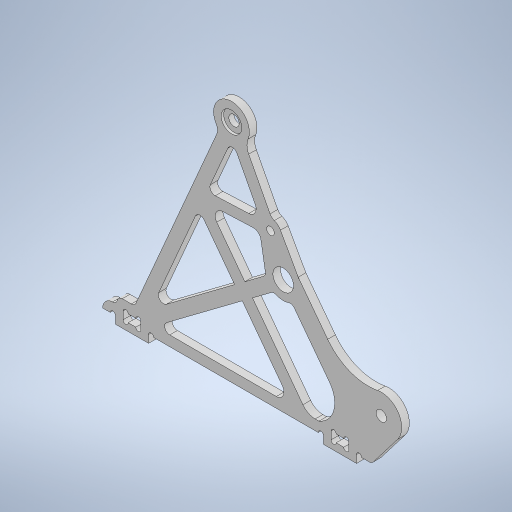
# Autodesk Inventor part: 左フレーム
Saved by Autodesk Inventor 2023 (Build 270158000, 158)
## iProperties
Created: 2022-04-10
Part Number: 左フレーム
Material: Generic
Document SubType Name: Modeling
Designer: acps
Density: 1 g/cm^3
Appearance: Default
Author: acps
Autodesk Inventor part; units mm, degrees
ref_plane "YZ Plane" through (0, 0, 0) normal (1, 0, 0) x (0, 1, 0)
ref_plane "XZ Plane" through (0, 0, 0) normal (0, 1, 0) x (-1, 0, 0)
ref_plane "XY Plane" through (0, 0, 0) normal (0, 0, 1) x (1, 0, 0)
sketch "Sketch1" plane through (0, 0, 0) normal (0, 0, 1) x (1, 0, 0)
  circle A0 centre (76.7566, -3) radius 1
  circle A1 centre (71.7566, -3) radius 1
  circle A2 centre (71.7566, -6) radius 1
  circle A3 centre (-4.7865, -3) radius 1
  circle A4 centre (-4.7865, -6) radius 1
  circle A5 centre (-9.7865, -6) radius 1
  circle A6 centre (-9.7865, -3) radius 1
  circle A7 centre (76.7566, -6) radius 1
  circle A8 centre (31.7211, 82.4471) radius 2.025
  circle A9 centre (31.7211, 82.4471) radius 7
  circle A10 centre (47, 53.101) radius 1.5
  circle A11 centre (52, 38.9589) radius 4.025
  circle A12 centre (52, 38.9589) radius 7.025
  circle A13 centre (47, 53.101) radius 4.5
  circle A14 centre (90.4665, 12.0244) radius 2.025
  circle A15 centre (66.7566, -6) radius 1
  circle A16 centre (81.7566, -6) radius 1
  line L0 (67.7566, -9) -> (80.7566, -9)
  line L1 (80.7566, -9) -> (80.7566, -6)
  line L2 (67.7566, -6) -> (67.7566, -9)
  circle A17 centre (-14.7865, -6) radius 1
  line L3 (-13.7865, -6) -> (-13.7865, -9)
  line L4 (-13.7865, -9) -> (-0.7865, -9)
  circle A18 centre (0.2135, -6) radius 1
  line L5 (-0.7865, -9) -> (-0.7865, -6)
  line L6 (72.7566, -3) -> (75.7566, -3)
  line L7 (70.7566, -3) -> (70.7566, -6)
  line L8 (77.7566, -3) -> (77.7566, -6)
  line L9 (72.7566, -6) -> (75.7566, -6)
  line L10 (67.7566, -6) -> (70.7566, -6)
  line L11 (77.7566, -6) -> (80.7566, -6)
  line L12 (1.2135, -6) -> (65.7566, -6)
  line L13 (-8.7865, -3) -> (-5.7865, -3)
  line L14 (-3.7865, -3) -> (-3.7865, -6)
  line L15 (-10.7865, -3) -> (-10.7865, -6)
  line L16 (-13.7865, -6) -> (-10.7865, -6)
  line L17 (-3.7865, -6) -> (-0.7865, -6)
  line L18 (-5.7865, -6) -> (-8.7865, -6)
  arc A19 (-14.9185, -2.0022) -> (-18.7865, -6) centre (-14.7865, -6) ccw
  line L19 (-15.7865, -6) -> (-18.7865, -6)
  arc A20 (-14.9185, -2.0022) -> (-13.0476, -0.5016) centre (-14.9845, -0.0033) ccw
  line L20 (-11.1107, 1) -> (-3.5008, 1)
  arc A21 (-11.1107, 1) -> (-13.0476, -0.5016) centre (-11.1107, -1) ccw
  arc A22 (-3.5008, 1) -> (-2.3017, 1.3994) centre (-3.5008, 3) ccw
  line L21 (-2.3017, 1.3994) -> (44.2402, 36.269)
  arc A23 (44.2402, 36.269) -> (45.0264, 38.111) centre (43.041, 37.8696) ccw
  line L22 (-7.2865, -3) -> (-7.2865, 1.4065) construction
  line L23 (1.2135, -6) -> (4.2135, -6)
  line L24 (3.5461, -0.4671) -> (47.2381, 32.2675)
  arc A24 (49.2268, 32.5044) -> (47.2381, 32.2675) centre (48.4373, 30.6668) ccw
  arc A25 (4.2135, -6) -> (3.2347, -3.3784) centre (0.2135, -6) ccw
  arc A26 (3.5461, -0.4671) -> (3.2347, -3.3784) centre (4.7453, -2.0677) ccw
  line L25 (0, 0) -> (52, 38.9589) construction
  arc A27 (6.3059, 1.6006) -> (7.5051, -2) centre (7.5051, 0) ccw
  line L26 (7.5051, -2) -> (66.0314, -2)
  arc A28 (65.458, -2.2167) -> (62.7566, -6) centre (66.7566, -6) ccw
  arc A29 (65.458, -2.2167) -> (70.1898, 13.2706) centre (62.2116, 7.2417) ccw
  line L27 (70.1898, 13.2706) -> (56.3591, 31.5732)
  line L28 (85.7566, -6) -> (82.7566, -6)
  circle A30 centre (90.4665, 12.0244) radius 8
  arc A31 (85.7566, -6) -> (87.3447, -5.2156) centre (85.7566, -4) ccw
  line L29 (87.3447, -5.2156) -> (96.8191, 7.1618)
  line L30 (57.6047, 43.1942) -> (69.4589, 27.5072)
  arc A32 (69.4589, 27.5072) -> (89.0233, 19.8931) centre (85.4154, 39.565) ccw
  arc A33 (56.3591, 31.5732) -> (54.1511, 32.2713) centre (54.7635, 30.3674) ccw
  arc A34 (3.1955, 10.1861) -> (6.2304, 7.7917) centre (5.0312, 9.3923) ccw
  line L31 (3.1955, 10.1861) -> (30.2617, 72.7739)
  arc A35 (-7.5387, 1) -> (-5.703, 2.2061) centre (-7.5387, 3) ccw
  line L32 (-5.703, 2.2061) -> (25.9041, 75.2943)
  line L33 (31.7211, 82.4471) -> (-3.5008, 1) construction
  arc A36 (59.7531, 0.4024) -> (68.07, -0.8626) centre (64.5549, 4) ccw
  line L34 (59.7531, 0.4024) -> (21.9068, 50.9174)
  line L35 (51.7101, 2.7988) -> (20.9924, 43.7989)
  arc A37 (20.9924, 43.7989) -> (17.5561, 43.3936) centre (19.3918, 42.5997) ccw
  arc A38 (21.6717, 52.9105) -> (21.9068, 50.9174) centre (23.5074, 52.1166) ccw
  arc A39 (49.3092, -2) -> (51.7101, 2.7988) centre (49.3092, 1) ccw
  line L36 (42.5654, 52.3366) -> (45.0771, 37.7656)
  line L37 (50.9296, 55.2938) -> (58.1345, 42.3821)
  arc A40 (33.8713, 72.9036) -> (30.2617, 72.7739) centre (32.0974, 71.98) ccw
  line L38 (33.8713, 72.9036) -> (42.6165, 56.1068)
  arc A41 (42.7371, 54.5426) -> (42.6165, 56.1068) centre (40.8425, 55.1832) ccw
  line L39 (31.7211, 82.4471) -> (47, 53.101) construction
  arc A42 (38.2267, 79.8629) -> (38.481, 74.8771) centre (43.8028, 77.6479) ccw
  line L40 (38.481, 74.8771) -> (46.8627, 58.7783)
  arc A43 (46.8627, 58.7783) -> (48.5142, 57.3386) centre (49.5237, 60.1637) ccw
  arc A44 (25.9041, 75.2943) -> (25.6831, 78.9057) centre (22.2327, 76.882) ccw
  arc A45 (23.435, 56.9879) -> (25.3544, 54.1958) centre (25.2707, 56.194) ccw
  line L41 (25.3544, 54.1958) -> (38.5073, 54.7469)
  arc A46 (38.5073, 54.7469) -> (41.0427, 59.1297) centre (38.3817, 57.7443) ccw
  arc A47 (28.2285, 50.3127) -> (25.9532, 45.5165) centre (28.3541, 47.3153) ccw
  line L42 (28.2285, 50.3127) -> (40.1748, 50.8133)
  arc A48 (43.2568, 48.3255) -> (40.1748, 50.8133) centre (40.3004, 47.8159) ccw
  line L43 (23.5074, 52.1166) -> (47, 53.101) construction
  circle A49 centre (31.7211, 82.4471) radius 4.03
  point P0 (36.9651, 30.8184)
  point P1 (45.0367, 37.9996)
  point P2 (39.9631, 26.8169)
  point P3 (64.5549, -2)
  point P4 (35.9616, 23.819)
  point P5 (57.8977, 42.8065)
  point P6 (32.9636, 27.8205)
  dimension "d54" = 4.05
  dimension "d55" = 14
  dimension "d56" = 3
  dimension "d57" = 8.05
  dimension "d58" = 3
  dimension "d59" = 3
  dimension "d60" = 4.05
  dimension "d61" = 3
  dimension "d62" = 2
  dimension "d63" = 3
  dimension "d64" = 2
  dimension "d65" = 3
  dimension "d66" = 2
  dimension "d67" = 2
  dimension "d68" = 2
  dimension "d69" = 2
  dimension "d70" = 3
  dimension "d71" = 5
  dimension "d72" = 2.5
  dimension "d73" = 2
  dimension "d74" = 4
  dimension "d75" = 3
  dimension "d76" = 10
  dimension "d77" = 3
  dimension "d78" = 16
  dimension "d79" = 2
  dimension "d80" = 20
  dimension "d81" = 2
  dimension "d82" = 8
  dimension "d83" = 2
  dimension "d84" = 2
  dimension "d85" = 5
  dimension "d86" = 2.5
  dimension "d87" = 6
  dimension "d88" = 2
  dimension "d89" = 2
  dimension "d90" = 5
  dimension "d91" = 3
  dimension "d92" = 2
  dimension "d93" = 2
  dimension "d94" = 6
  dimension "d95" = 3
  dimension "d96" = 5
  dimension "d97" = 2.5
  dimension "d98" = 4
  dimension "d99" = 3
  dimension "d100" = 2
  dimension "d101" = 3
  dimension "d102" = 3
  dimension "d103" = 3
  dimension "d104" = 4
  dimension "d105" = 2
  dimension "d106" = 8.06
  constraints: 94 point on circle, 88 end point, 62 tangent, 50 centre point, 18 point on line, 11 parallel, 10 horizontal, 7 coincident, 5 vertical, 4 horizontal alignment, 3 collinear, 3 concentric, 3 perpendicular, 1 midpoint, 1 symmetric about line, 17 other
  measures "d54" diameter of A8
  measures "d55" diameter of A9
  measures "d56" diameter of A10
  measures "d57" diameter of A11
  measures "d58" radial gap between concentric circles of A11 A12
  measures "d59" radial gap between concentric circles of A10 A13
  measures "d60" diameter of A14
  measures "d61" radial gap between concentric circles of A17 A19
  measures "d62" radius of A20
  measures "d63" distance edge to line of A6 L20
  measures "d64" radius of A21
  measures "d66" radius of A22
  measures "d67" radius of A23
  measures "d68" radius of A24
  measures "d69" radius of A26
  measures "d70" radial gap between concentric circles of A18 A25
  measures "d71" distance between parallel lines of L24 L21
  measures "d72" distance between parallel lines of L25 L21
  measures "d73" radius of A27
  measures "d74" distance between parallel lines of L12 L26
  measures "d75" radial gap between concentric circles of A28 A15
  measures "d76" radius of A29
  measures "d78" diameter of A30
  measures "d79" radius of A31
  measures "d80" radius of A32
  measures "d81" radius of A33
  measures "d82" distance between parallel lines of L27 L30
  measures "d83" radius of A34
  measures "d84" radius of A35
  measures "d85" distance between parallel lines of L32 L31
  measures "d86" distance between parallel lines of L32 L33
  measures "d87" radius of A36
  measures "d88" radius of A37
  measures "d89" radius of A38
  measures "d90" distance between parallel lines of L35 L34
  measures "d91" radius of A39
  measures "d92" radius of A40
  measures "d93" radius of A41
  measures "d94" radius of A42
  measures "d95" radius of A43
  measures "d96" distance between parallel lines of L38 L40
  measures "d97" distance between parallel lines of L38 L39
  measures "d98" radius of A44
  measures "d99" distance of L28.start L28.end
  measures "d100" radius of A45
  measures "d101" radius of A46
  measures "d102" radius of A47
  measures "d103" radius of A48
  measures "d104" distance between parallel lines of L42 L41
  measures "d105" distance between parallel lines of L41 L43
  measures "d106" diameter of A49
extrude "Extrusion1" add sketch "Sketch1" along normal blind 3 contours A0 L6 A1 L7 L10 A15 L12 A28 A29 L27 A33 A12 L37 L30 A32 A30 L29 A31 L28 A16 L11 L8 | L11 L1 L0 L2 L10 A2 L9 A7 | A30 | L12 A25 A26 L24 A27 L26 A29 A28 | L12 A18 L17 L14 A3 L13 A6 L15 L16 A17 L19 A19 A20 A21 L20 A22 L21 L35 L24 A26 A25 | L30 A12 A23 L36 A13 L37 | L5 L4 L3 L16 A5 L18 A4 L17 | L26 A39 L35 L24 L34 A36 | A12 | A13 | A13 A41 L38 A40 L31 A34 L21 A22 L20 A35 L32 A44 A9 A42 L40 A43 | L35 L21 L34 L24 | L34 L21 A23 L36 A12 A24 L24 | L36 A48 L42 A47 L34 A38 L31 A45 L41 A46 L38 A41 A13 | L35 A37 L31 A38 L34 L21 | A9
extrude "Extrusion2" add sketch "Sketch1" along normal blind 2 contours A49
equation "\"d72\" = 0.5 * d71"
equation "\"d86\" = 0.5 * d85"
equation "\"d97\" = 0.5 * d96"
equation "\"d105\" = 0.5 * d104"
body "Solid1"
